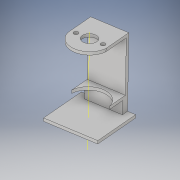
# Autodesk Inventor part: motor connector
Saved by Autodesk Inventor 2019 (Build 230136000, 136)
## iProperties
Created: 2020-03-18
Part Number: motor connector
Material: Generic
Document SubType Name: Modeling
Designer: 18186
Density: 1 g/cm^3
Appearance: Default
Author: 18186
Autodesk Inventor part; units mm, degrees
ref_plane "YZ Plane" through (0, 0, 0) normal (1, 0, 0) x (0, 1, 0)
ref_plane "XZ Plane" through (0, 0, 0) normal (0, 1, 0) x (-1, 0, 0)
ref_plane "XY Plane" through (0, 0, 0) normal (0, 0, 1) x (1, 0, 0)
sketch "Sketch1" plane through (0, 0, 0) normal (0, 0, 1) x (1, 0, 0)
  line L0 (-9.4319, 10.8445) -> (26.5681, 10.8445)
  line L1 (26.5681, 10.8445) -> (26.5681, -46.1555)
  line L2 (26.5681, -46.1555) -> (-9.4319, -46.1555)
  line L3 (-9.4319, -46.1555) -> (-9.4319, 10.8445)
  point P0 (0, 0)
  dimension "d0" = 36
  dimension "d1" = 57
  constraints: 8 end point, 2 parallel, 1 horizontal, 1 perpendicular
  measures "d0" distance of L1.end L2.end
  measures "d1" distance of L0.end L1.end
extrude "Extrusion1" add sketch "Sketch1" along normal blind 3
sketch "Sketch2" plane through (-9.4319, 10.8445, 0) normal (0, 1, 0) x (1, 0, 0)
  line L0 (0, 0) -> (36, 0) construction
  line L1 (0, -3) -> (0, -22.268)
  line L2 (36, -3) -> (36, -22.268)
  line L3 (18, 0) -> (18, -6.949) construction
  arc A0 (36, -22.268) -> (0, -22.268) centre (18, -25.1836) ccw
  line L4 (36, -3) -> (0, -3) projected
  line L5 (36, -3) -> (0, -3)
  point P0 (9.4319, 0)
  dimension "d4" = 22.268
  dimension "d5" = 6.949
  constraints: 8 end point, 3 point on circle, 3 vertical, 2 point on line, 1 centre point, 1 collinear, 1 midpoint
  measures "d4" distance of L0.start L1.end
  measures "d5" distance of L3.start L3.end
extrude "Extrusion2" add sketch "Sketch2" against normal blind 3
sketch "Sketch3" plane through (-9.4319, -46.1555, 0) normal (0, -1, 0) x (1, 0, 0)
  line L0 (0, 0) -> (0, 22.268) construction
  line L1 (36, 0) -> (36, 22.268) construction
  arc A0 (36, 28.0992) -> (0, 28.0992) centre (18, 25.1836) ccw
  line L2 (0, 22.268) -> (0, 28.0992)
  line L3 (36, 22.268) -> (36, 28.0992)
  line L4 (0, 3) -> (36, 3) projected
  arc A1 (0, 22.268) -> (36, 22.268) centre (18, 25.1836) ccw construction
  line L5 (0, 3) -> (0, 22.268)
  line L6 (36, 3) -> (36, 22.268)
  line L7 (0, 3) -> (36, 3)
  point P0 (9.4319, 0)
  constraints: 10 end point, 3 point on circle, 2 collinear, 2 vertical, 1 centre point, 1 point on line
extrude "Extrusion3" add sketch "Sketch3" against normal blind 3
sketch "Sketch4" plane through (-9.4319, -46.1555, 0) normal (0, -1, 0) x (1, 0, 0)
  line L0 (0, 0) -> (36, 0) projected
  line L1 (18, 0) -> (18, 17.95) construction
  line L2 (18, 17.95) -> (18, 24.95) construction
  circle A0 centre (18, 24.95) radius 7
  line L3 (7.486, 24.95) -> (5.236, 24.95) construction
  circle A1 centre (5.236, 24.95) radius 2.25
  circle A2 centre (30.764, 24.95) radius 2.25
  point P0 (9.4319, 0)
  dimension "d10" = 17.95
  dimension "d11" = 7
  dimension "d13" = 2.25
  constraints: 6 end point, 2 coincident, 1 centre point, 1 horizontal, 1 horizontal alignment, 1 midpoint, 1 point on line, 1 symmetric about line, 1 vertical, 1 vertical alignment, 5 other
  measures "d10" distance of L1.start L1.end
  measures "d11" distance of L1.end L2.end
  measures "d13" distance of L3.start L3.end
extrude "Extrusion4" cut sketch "Sketch4" against normal blind 3
sketch "Sketch5" plane through (-9.4319, 10.8445, 0) normal (0, 1, 0) x (1, 0, 0)
  line L0 (36, 0) -> (0, 0) projected
  line L1 (36, 0) -> (36, -28.0992) projected
  line L2 (0, 0) -> (36, 0)
  line L3 (36, 0) -> (36, -6.35)
  line L4 (36, -6.35) -> (0, -6.35)
  line L5 (0, -6.35) -> (0, 0)
  point P0 (9.4319, 0)
  dimension "d17" = 6.35
  constraints: 8 end point, 2 parallel, 1 horizontal, 1 perpendicular, 1 point on line
  measures "d17" distance of L2.end L3.end
extrude "Extrusion5" add sketch "Sketch5" along normal blind 12.7
sketch "Sketch6" plane through (-9.4319, 23.5445, 0) normal (0, 1, 0) x (1, 0, 0)
  line L0 (43.62, 0) -> (-7.62, 0)
  line L1 (-7.62, 0) -> (-7.62, -46.7504)
  line L2 (-7.62, -46.7504) -> (43.62, -46.7504)
  line L3 (43.62, -46.7504) -> (43.62, 0)
  line L4 (36, 0) -> (36, -28.0992) projected
  line L5 (0, 0) -> (0, -28.0992) projected
  dimension "d22" = 7.62
  dimension "d23" = 7.62
  constraints: 8 end point, 2 parallel, 1 horizontal, 1 perpendicular
  measures "d22" distance between parallel lines of L3 L4
  measures "d23" distance between parallel lines of L5 L1
extrude "Extrusion6" add sketch "Sketch6" along normal blind 3
body "Solid1"
